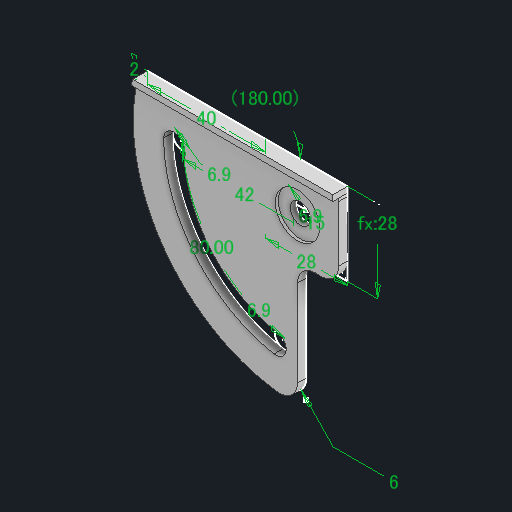
# Autodesk Inventor part: baicPart
Saved by Autodesk Inventor 2025.2 (Build 292293000, 293)
## iProperties
Company: FC-TORQUE
Created: 2025-03-14
Part Number: baicPart
Material: 一般
Document SubType Name: Modeling
Designer: Keito Tamura
Density: 1 g/cm^3
Appearance: 既定
Author: Keito Tamura
Autodesk Inventor part; units mm, degrees
ref_plane "YZ Plane" through (0, 0, 0) normal (1, 0, 0) x (0, 1, 0)
ref_plane "XZ Plane" through (0, 0, 0) normal (0, 1, 0) x (-1, 0, 0)
ref_plane "XY Plane" through (0, 0, 0) normal (0, 0, 1) x (1, 0, 0)
sketch "スケッチ1" plane through (0, 0, 0) normal (0, 0, 1) x (1, 0, 0)
  circle A0 centre (0, 0) radius 3.45
  circle A1 centre (0, 0) radius 7.5
  line L0 (-14, 14) -> (14, 14)
  line L1 (14, 14) -> (14, -14)
  line L2 (14, -14) -> (-14, -14)
  line L3 (-14, -14) -> (-14, 14)
  line L4 (-14, 14) -> (14, -14) construction
  line L5 (14, 14) -> (-14, -14) construction
  line L6 (-14, 14) -> (-54, 14)
  line L7 (-14, 14) -> (26, 14) construction
  arc A2 (-54, 14) -> (-6.7231, -55.3787) centre (0, 0) ccw
  line L8 (0, 0) -> (-42, 0)
  circle A3 centre (-42, 0) radius 3.45
  line L9 (0, -14) -> (0, -49.4224)
  circle A4 centre (-7.2932, -41.3619) radius 3.45
  arc A5 (-38.55, 0) -> (-6.6941, -37.9643) centre (0, 0) ccw
  arc A6 (-45.45, 0) -> (-7.301, -44.8598) centre (0, 0) ccw
  arc A7 (-6.7231, -55.3787) -> (0, -49.4224) centre (-6, -49.4224) ccw
  line L10 (14, 12) -> (-54.4794, 12)
  point P0 (0, -55.7853)
  point P1 (-7.8923, -44.7595)
  dimension "d0" = 6.9
  dimension "d1" = 15
  dimension "d2" = 28
  dimension "d3" = 28
  dimension "d8" = 40
  dimension "d9" = 180
  dimension "d10" = 42
  dimension "d11" = 6.9
  dimension "d14" = 80
  dimension "d16" = 6.9
  dimension "d17" = 6
  dimension "d23" = 2
  constraints: 22 end point, 12 point on circle, 7 centre point, 6 coincident, 5 horizontal, 3 midpoint, 3 point on line, 2 parallel, 2 tangent, 1 collinear, 1 perpendicular, 1 vertical, 6 other
  measures "d0" diameter of A0
  measures "d1" diameter of A1
  measures "d2" distance of L1.end L2.end
  measures "d3" distance of L0.end L1.end
  measures "d8" distance of L0.start L6.end
  measures "d9" angle of L6 L7
  measures "d10" distance of L8.start L8.end
  measures "d11" diameter of A3
  measures "d16" radial gap between concentric circles of A5 A6
  measures "d17" radius of A7
  measures "d23" distance between parallel lines of L6 L10
extrude "押し出し1" add sketch "スケッチ1" along normal blind 3 contours L0 L1 L10 L3 | L10 L1 L2 L3
extrude "押し出し2" add sketch "スケッチ1" along normal blind 2 contours A1
extrude "押し出し3" add sketch "スケッチ1" along normal blind 3 contours L3 L10 A2 L6 | L3 L2 L9 A7 A2 L10
fillet "フィレット1" radius 6 2 edges at (14, -14, 1.5) (0, -14, 1.5)
fillet "フィレット2" radius 3 1 edges at (14, 14, 1.5)
fillet "フィレット3" radius 2 1 edges at (-54, 14, 1.5)
extrude "押し出し4" add sketch "スケッチ1" along normal blind 5 contours L0 L1 L10 L3 | L3 L10 A2 L6
equation "\"d3\" = d2"
